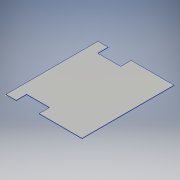
# Autodesk Inventor part: Belly Pan
Saved by Autodesk Inventor 2018 (Build 220112000, 112)
## iProperties
Created: 2018-01-27
Part Number: Belly Pan
Material: Aluminum 6061
Document SubType Name: Modeling
Designer: s-4000369
Density: 2.7 g/cm^3
Appearance: Aluminum - Flat
Mass: 1648.73 g
Surface Area: 4866.5 cm^2
Volume: 610.641 cm^3
Author: s-4000369
Autodesk Inventor part; units mm, degrees
ref_plane "YZ Plane" through (0, 0, 0) normal (1, 0, 0) x (0, 1, 0)
ref_plane "XZ Plane" through (0, 0, 0) normal (0, 1, 0) x (-1, 0, 0)
ref_plane "XY Plane" through (0, 0, 0) normal (0, 0, 1) x (1, 0, 0)
sketch "Sketch1" plane through (0, 0, 0) normal (0, 1, 0) x (-1, 0, 0)
  point P0 (0, 0)
sketch "Sketch2" plane through (0, 0, 0) normal (0, 1, 0) x (-1, 0, 0)
  line L0 (-61.9252, 0) -> (0, 0)
  line L1 (0, 0) -> (0, -558.8)
  line L2 (0, -558.8) -> (-61.9252, -558.8)
  line L3 (-61.9252, -558.8) -> (-61.9252, -495.3)
  line L4 (-61.9252, -495.3) -> (-201.6252, -495.3)
  line L5 (-201.6252, -495.3) -> (-201.6252, -558.8)
  line L6 (-201.6252, -558.8) -> (-461.9752, -558.8)
  line L7 (-461.9752, -558.8) -> (-461.9752, 0)
  line L8 (-461.9752, 0) -> (-201.6252, 0)
  line L9 (-201.6252, 0) -> (-201.6252, -63.5)
  line L10 (-201.6252, -63.5) -> (-61.9252, -63.5)
  line L11 (-61.9252, -63.5) -> (-61.9252, 0)
  point P0 (0, 0)
  dimension "d1" = 558.8
  dimension "d2" = 139.7
  dimension "d3" = 61.9252
  dimension "d4" = 63.5
  dimension "d8" = 260.35
  constraints: 24 end point, 8 perpendicular, 5 point on line, 2 collinear, 1 coincident, 1 horizontal, 1 vertical
  measures "d1" distance between parallel lines of L6 L8
  measures "d2" distance of L9.end L10.end
  measures "d3" distance of L0.start L0.end
  measures "d4" distance of L8.end L9.end
  measures "d8" distance of L7.end L8.end
extrude "Extrusion1" add sketch "Sketch2" along normal blind 2.54
body "Solid1"
